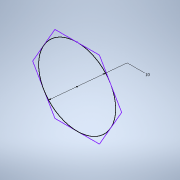
# Autodesk Inventor part: 18_Vite_M6_L100
Saved by Autodesk Inventor 2020 (Build 240168000, 168)
## iProperties
Created: 2019-10-18
Part Number: 18_Vite_M6_L100
Material: Generico
Document SubType Name: Modeling
Designer: socci
Density: 1 g/cm^3
Appearance: Default
Author: socci
Autodesk Inventor part; units mm, degrees
ref_plane "YZ Plane" through (0, 0, 0) normal (1, 0, 0) x (0, 1, 0)
ref_plane "XZ Plane" through (0, 0, 0) normal (0, 1, 0) x (-1, 0, 0)
ref_plane "XY Plane" through (0, 0, 0) normal (0, 0, 1) x (1, 0, 0)
sketch "Schizzo1" plane through (0, 0, 0) normal (0, 0, 1) x (1, 0, 0)
  circle A0 centre (0, 0) radius 5
  line L0 (2.8868, 5) -> (5.7735, 0)
  line L1 (5.7735, 0) -> (2.8868, -5)
  line L2 (2.8868, -5) -> (-2.8868, -5)
  line L3 (-2.8868, -5) -> (-5.7735, 0)
  line L4 (-5.7735, 0) -> (-2.8868, 5)
  line L5 (-2.8868, 5) -> (2.8868, 5)
  point P0 (0, 5)
  dimension "d0" = 10
  constraints: 12 end point, 2 coincident, 1 midpoint, 1 vertical alignment, 15 other
extrude "Estrusione1" add sketch "Schizzo1" along normal blind 4
sketch "Schizzo3" plane through (0, 0, 0) normal (0, 0, -1) x (-1, 0, 0)
  circle A0 centre (0, 0) radius 3
  dimension "d3" = 6
  constraints: 1 centre point, 1 coincident
  measures "d3" diameter of A0
extrude "Estrusione2" add sketch "Schizzo3" along normal blind 100
thread "Filettatura1" size "M6x1" class "6g" standard "ANSI Metric M Profile" full length
fillet "Raccordo1" radius 1 1 edges at (3, 0, -100)
